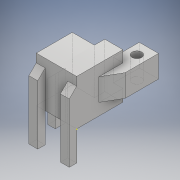
# Autodesk Inventor part: Y- motor carrier
Saved by Autodesk Inventor 2018 (Build 220112000, 112)
## iProperties
Created: 2018-04-19
Part Number: Y- motor carrier
Material: Generic
Document SubType Name: Modeling
Designer: junai
Density: 1 g/cm^3
Appearance: Default
Mass: 30.5506 g
Surface Area: 86.1677 cm^2
Volume: 30.5506 cm^3
Author: junai
Autodesk Inventor part; units mm, degrees
ref_plane "YZ Plane" through (0, 0, 0) normal (1, 0, 0) x (0, 1, 0)
ref_plane "XZ Plane" through (0, 0, 0) normal (0, 1, 0) x (-1, 0, 0)
ref_plane "XY Plane" through (0, 0, 0) normal (0, 0, 1) x (1, 0, 0)
sketch "Sketch1" plane through (0, 0, 0) normal (0, 1, 0) x (-1, 0, 0)
  line L0 (0, 0) -> (27.3, 0)
  line L1 (27.3, 0) -> (27.3, -30.7)
  line L2 (27.3, -30.7) -> (0, -30.7)
  line L3 (0, -30.7) -> (0, 0)
  dimension "d0" = 27.3
  dimension "d1" = 30.7
  constraints: 8 end point, 2 parallel, 1 horizontal, 1 perpendicular
  measures "d0" distance of L1.end L2.end
  measures "d1" distance of L0.end L1.end
extrude "Extrusion1" add sketch "Sketch1" along normal blind 31.3
sketch "Sketch2" plane through (0, 31.3, 0) normal (0, 1, 0) x (1, 0, 0)
  line L0 (-27.3, 0) -> (0, 0) construction
  line L1 (0, 0) -> (0, 7.7) construction
  line L2 (-6.5, 7.7) -> (6.5, 7.7)
  line L3 (6.5, 7.7) -> (6.5, 22.7)
  line L4 (6.5, 22.7) -> (-6.5, 22.7)
  line L5 (-6.5, 22.7) -> (-6.5, 7.7)
  dimension "d4" = 7.7
  dimension "d5" = 13
  dimension "d6" = 15
  constraints: 10 end point, 2 parallel, 1 horizontal, 1 midpoint, 1 perpendicular, 1 vertical
  measures "d4" distance of L1.end L0.end
  measures "d5" distance of L4.end L3.end
  measures "d6" distance of L4.end L2.start
extrude "Extrusion2" add sketch "Sketch2" along normal blind 20 and the other way blind 5
draft "FaceDraft1" angle 60 pull direction (1, 0, 0) faces at (2.1667, 26.3, -17.7) fixed edges at (6.5, 26.3, -15.2)
sketch "Sketch3" plane through (-6.5, 31.3, -7.7) normal (0, 0, 1) x (1, 0, 0)
  line L0 (6.5, 0) -> (0, 0) construction
  line L1 (0, 0) -> (0, 6.2) construction
  line L2 (0, 20) -> (0, 0) construction
  line L3 (0, 6.2) -> (12.9928, 6.2) construction
  circle A0 centre (6.4964, 9.425) radius 3.225
  line L4 (0, 20) -> (13, 20) projected
  line L5 (0, 20) -> (13, 20)
  line L6 (13, 20) -> (13, 17.5)
  line L7 (13, 17.5) -> (0, 17.5)
  line L8 (0, 17.5) -> (0, 20)
  point P0 (6.5, -31.3)
  point P1 (6.4964, 6.2)
  dimension "d13" = 6.45
  dimension "d12" = 6.2
  dimension "d14" = 2.5
  constraints: 12 end point, 3 horizontal, 2 parallel, 1 midpoint, 1 perpendicular, 1 point on line, 1 vertical alignment, 2 other
  measures "d12" distance of L0.end L1.end
  measures "d14" distance between parallel lines of L4 L7
extrude "Extrusion3" cut sketch "Sketch3" against normal through all
sketch "Sketch4" plane through (0, 0, -30.7) normal (0, 0, -1) x (-1, 0, 0)
  line L0 (27.3, 31.3) -> (0, 31.3) construction
  line L1 (27.3, 31.3) -> (27.3, 19.8) construction
  line L2 (27.3, 0) -> (27.3, 31.3) construction
  line L3 (27.3, 19.8) -> (32.3, 19.8)
  line L4 (32.3, 19.8) -> (32.3, 12.8)
  line L5 (32.3, 12.8) -> (27.3, 12.8)
  line L6 (27.3, 12.8) -> (27.3, 19.8)
  point P0 (0, 0)
  dimension "d17" = 11.5
  dimension "d18" = 5
  dimension "d19" = 7
  constraints: 10 end point, 2 parallel, 1 horizontal, 1 perpendicular, 1 point on line
  measures "d17" distance of L0.start L1.end
  measures "d18" distance of L4.end L5.end
  measures "d19" distance of L3.end L4.end
extrude "Extrusion4" add sketch "Sketch4" along normal blind 20 and the other way blind 12
draft "FaceDraft2" angle 45 pull direction (-1, 0, 0) faces at (-30.6333, 15.1333, -18.7) fixed edges at (-27.3, 16.3, -18.7)
sketch "Sketch5" plane through (0, 0, -30.7) normal (0, 0, -1) x (-1, 0, 0)
  line L0 (27.3, 19.8) -> (27.3, 31.3) projected
  line L1 (27.3, 31.3) -> (12.3, 31.3)
  line L2 (12.3, 31.3) -> (12.3, 24.3)
  line L3 (12.3, 24.3) -> (27.3, 24.3)
  line L4 (27.3, 24.3) -> (27.3, 31.3)
  point P0 (0, 0)
  dimension "d25" = 15
  dimension "d26" = 7
  constraints: 8 end point, 2 parallel, 1 horizontal, 1 perpendicular
  measures "d25" distance of L3.end L2.end
  measures "d26" distance between parallel lines of L3 L1
extrude "Extrusion5" cut sketch "Sketch5" against normal through all
sketch "Sketch6" plane through (0, 0, -30.7) normal (0, 0, -1) x (-1, 0, 0)
  point P0 (0, 0)
sketch "Sketch7" plane through (0, 0, -30.7) normal (0, 0, -1) x (-1, 0, 0)
  point P0 (0, 0)
sketch "Sketch8" plane through (0, 0, -30.7) normal (0, 0, -1) x (-1, 0, 0)
  line L0 (27.3, 0) -> (0, 0) projected
  line L1 (27.3, 0) -> (21.3, 0)
  line L2 (21.3, 0) -> (21.3, -5)
  line L3 (21.3, -5) -> (27.3, -5)
  line L4 (27.3, -5) -> (27.3, 0)
  line L5 (0, 0) -> (6, 0)
  line L6 (6, 0) -> (6, -5)
  line L7 (6, -5) -> (0, -5)
  line L8 (0, -5) -> (0, 0)
  dimension "d29" = 6
  dimension "d30" = 5
  dimension "d31" = 6
  dimension "d32" = 5
  constraints: 16 end point, 4 parallel, 2 horizontal, 2 perpendicular
  measures "d29" distance of L3.end L2.end
  measures "d30" distance of L1.end L2.end
  measures "d31" distance of L6.end L7.end
  measures "d32" distance of L7.end L0.end
extrude "Extrusion6" add sketch "Sketch8" along normal blind 20 and the other way blind 25
draft "FaceDraft3" angle 45 pull direction (0, -1, 0) faces at (-23.3, -3.3333, -5.7) (-2, -1.6667, -5.7) fixed edges at (-24.3, 0, -5.7) (-3, 0, -5.7)
body "Solid1"
